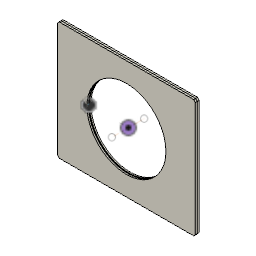
Condensor lens mount (Autodesk Fusion 360 design; units mm, degrees)
part number: 2026-06-29-18-31-42-518
Autodesk Fusion 360 part; units mm, degrees
sketch "Sketch1" plane through (0, 0, 0) normal (0, 1, 0) x (1, 0, 0)
  line L0 (87.5, -75) -> (-87.5, -75)
  line L1 (-87.5, -75) -> (-87.5, 75)
  line L2 (-87.5, 75) -> (87.5, 75)
  line L3 (87.5, 75) -> (87.5, -75)
  line L4 (87.5, -75) -> (-87.5, 75) construction
  line L5 (-87.5, -75) -> (87.5, 75) construction
  line L6 (-87.5, -72.7222) -> (-85.5476, -75)
  line L7 (0, -75) -> (0, 75) construction
  line L8 (-87.5, 0) -> (87.5, 0) construction
  line L9 (87.5, -72.7222) -> (85.5476, -75)
  line L10 (87.5, 72.7222) -> (85.5476, 75)
  line L11 (-87.5, 72.7222) -> (-85.5476, 75)
  circle A0 centre (0, 0) radius 50
  dimension "d1" = 175
  dimension "d2" = 150
  dimension "d3" = 3
  dimension "d4" = 100
  constraint horizontal L0
  constraint perpendicular L0 L1
  constraint parallel L0 L2
  constraint parallel L1 L3
  constraint coincident L4 A0.centre
  constraint coincident L5 A0.centre
  constraint coincident A0.centre origin
  constraint coincident L1 L6.start
  constraint coincident L0 L6.end
  constraint perpendicular L5 L6
  constraint midpoint L0 L7.start
  constraint midpoint L2 L7.end
  constraint midpoint L1 L8.start
  constraint midpoint L3 L8.end
  constraint symmetric L6.start L7 L9.start
  constraint symmetric L6.end L7 L9.end
  constraint symmetric L6.start L8 L11.start
  constraint symmetric L6.end L8 L11.end
  constraint symmetric L8 L9.start L10.start
  constraint symmetric L8 L9.end L10.end
  measures "d1" distance of L1.end L2.end
  measures "d2" distance of L0.end L1.end
  measures "d3" distance of L6.start L6.end
  measures "d4" diameter of A0
sketch "Sketch2" plane through (0, 2.5, 0) normal (0, 1, 0) x (1, 0, 0)
sketch "Sketch3" plane through (50, 2.5597, 0) normal (-1, 0, 0) x (0, -1, 0)
sketch "Sketch5" plane through (0, 0, 0) normal (0, 0, 1) x (1, 0, 0)
  line L0 (-50, 0.5) -> (-50, -0.5)
  arc A0 (-50, 0.5) -> (-50, -0.5) centre (-50, 0) ccw
  line L1 (0, 20) -> (0, -21)
  line L2 (-50.5, 0) -> (0, 0) construction
  dimension "d9" = 1
  dimension "d14" = 1
  constraint vertical L0
  constraint midpoint L0 A0.centre
  constraint vertical L1
  constraint midpoint A0 L2.start
  constraint coincident L2.end origin
  constraint perpendicular L1 L2
  measures "d9" distance of L0.start L0.end
  measures "d14" diameter of A0
extrude "Extrude4" add sketch "Sketch1" along normal mid plane 5 contours L0 L1 L2 L3 L6 L9 L10 L11 makes body 1
revolve "Revolve2" cut sketch "Sketch5" angle 360 about axis through (0, 20, 0) along (0, -1, 0) bodies 1
fillet "Fillet1" radius 0.1 2 edges at (-46.6164, 0.5, -18.0808) (-46.6164, -0.5, 18.0808) on bodies 1
split "Split1" by plane through (0, 0, 0) normal (0, 1, 0) bodies 1 makes body 2 at (75, 2.5, 0)
